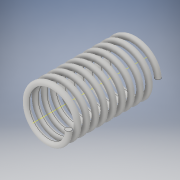
# Autodesk Inventor part: 示範四
Saved by Autodesk Inventor 2017 (Build 210142000, 142)
## iProperties
Part Number: 示範四
Material: 一般
Document SubType Name: Modeling
Designer: user
Density: 1 g/cm^3
Appearance: 預設
Author: user
Autodesk Inventor part; units mm, degrees
ref_plane "YZ Plane" through (0, 0, 0) normal (1, 0, 0) x (0, 1, 0)
ref_plane "XZ Plane" through (0, 0, 0) normal (0, 1, 0) x (-1, 0, 0)
ref_plane "XY Plane" through (0, 0, 0) normal (0, 0, 1) x (1, 0, 0)
sketch "草圖2" plane through (0, 0, 0) normal (0, 1, 0) x (-1, 0, 0)
  circle A0 centre (-13, 0) radius 1.5
  point P0 (0, 0)
  dimension "d1" = 3
  dimension "d2" = 13
  constraints: 1 centre point, 1 horizontal alignment
  measures "d1" diameter of A0
  measures "d2" distance of point (0, 0) A0.centre
coil "螺旋1" sketch "草圖2" operation add axis through (0, 0, -10) along (0, 0, 1) pitch 5 turns 10 hand right
